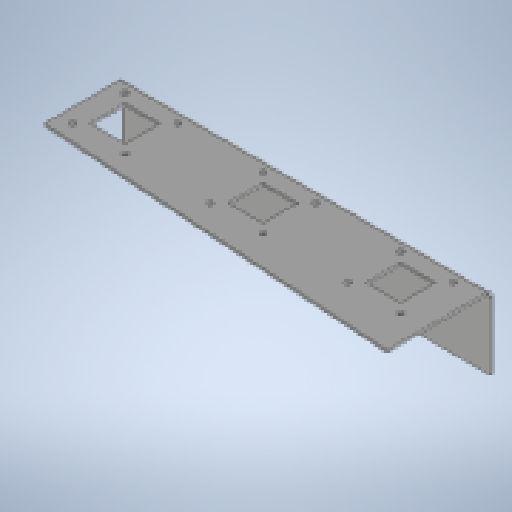
# Autodesk Inventor part: SLM 1422 BOTTOM FDS diameter way up
Saved by Autodesk Inventor 2026.2 (Build 302298000, 298)
## iProperties
Created: 2024-12-09
Part Number: SLM 1422 BOTTOM FDS diameter way up
Material: Stainless Steel
Document SubType Name: Sheet Metal
Designer: user
Mass: 793.765 g
Surface Area: 1023.32 cm^2
Volume: 99.2206 cm^3
Density: 8 g/cm^3
Flat Pattern Width: 15.2202 cm
Flat Pattern Length: 32 cm
Flat Pattern Area: 487.046 cm^2
Sheet Metal Rule: AISI304 2mm Die16
Sheet Metal Width: 152,202 mm
Sheet Metal Length: 320,000 mm
Sheet Metal Area: 48704,637 mm^2
Appearance: Default
Main_way_hight: 100,000 mm
Main_way_lenth: 410,000 mm
Small_ways_cross_H: 30,000 mm
Small_ways_cross_W: 30,000 mm
Author: user
Autodesk Inventor part; units mm, degrees
ref_plane "YZ Plane" through (0, 0, 0) normal (1, 0, 0) x (0, 1, 0)
ref_plane "XZ Plane" through (0, 0, 0) normal (0, 1, 0) x (-1, 0, 0)
ref_plane "XY Plane" through (0, 0, 0) normal (0, 0, 1) x (1, 0, 0)
sketch "Sketch1" plane through (0, 0, 0) normal (0, 0, 1) x (1, 0, 0)
  line L0 (0, 0) -> (-320, 0)
  line L1 (0, -92) -> (0, 0)
  line L2 (-320, 0) -> (-320, -70)
  line L3 (-320, -70) -> (0, -92)
  point P0 (0, -46)
  dimension "d32" = 92
  dimension "d60" = 70
  dimension "d61" = 320
  measures "d32" distance of L1.start L0.start
  measures "d60" distance of L0.end L2.end
  measures "d61" distance between parallel lines of L1 L2
extrude "Plate1" add sketch "Sketch1" along normal blind 2
sketch "Sketch8" plane through (0, 0, 2) normal (0, 0, 1) x (1, 0, 0)
  line L0 (-29.75, -50.25) -> (-60.25, -50.25)
  line L1 (-60.25, -50.25) -> (-60.25, -19.75)
  line L2 (-60.25, -19.75) -> (-29.75, -19.75)
  line L3 (-29.75, -19.75) -> (-29.75, -50.25)
  line L4 (-29.75, -50.25) -> (-60.25, -19.75) construction
  line L5 (-60.25, -50.25) -> (-29.75, -19.75) construction
  circle A0 centre (-22, -58) radius 2.5
  circle A1 centre (-68, -58) radius 2.5
  circle A2 centre (-68, -12) radius 2.5
  circle A3 centre (-22, -12) radius 2.5
  line L6 (0, 0) -> (0, -92) projected
  line L7 (-320, 0) -> (0, 0) projected
  line L8 (-60.25, -50.25) -> (-68, -58) construction
  line L9 (-68, -12) -> (-22, -12) construction
  line L10 (-22, -12) -> (-22, -58) construction
  line L11 (-22, -58) -> (-68, -58) construction
  line L12 (-68, -58) -> (-68, -12) construction
  point P0 (-45, -35)
  dimension "d51" = 30.5
  dimension "d52" = 30.5
  dimension "d53" = 5
  dimension "d72" = 45
  dimension "d78" = 46
  dimension "d79" = 12
  constraints: 22 end point, 4 centre point, 4 parallel, 4 point on line, 3 equal radius, 2 horizontal, 2 midpoint, 2 perpendicular
  measures "d51" distance of L0.start L0.end
  measures "d52" distance of L0.end L1.end
  measures "d53" diameter of A0
  measures "d72" distance from line of L6 point (-45, -35)
  measures "d78" distance of L8.end L9.start
  measures "d79" distance between parallel lines of L9 L7
extrude "Cut3" cut sketch "Sketch8" against normal blind 2
pattern_linear "Rectangular Pattern1" count 3 spacing 120 along (-1, 0, 0) of "Cut3"
sketch "Sketch9" plane through (0, -2, 2) normal (0, 1, 0) x (-1, 0, 0)
  line L0 (320, 0) -> (0, 0)
  line L1 (0, 0) -> (0, -64)
  line L2 (0, -64) -> (320, -64)
  line L3 (320, -64) -> (320, 0)
  constraints: 6 end point, 1 horizontal, 1 perpendicular, 1 vertical
edge flange "Flange3" height 64 angle 90 thickness 2 bend radius 2.75 thickness toward (0, 1, 0) relief round relief width 2 relief depth 1 edges at (-160, 0, 0) wall of the first edge with corners at (-320, -2, 2) (0, -2, 2) (0, -2, -62) (-320, -2, -62)
bend "Bend3"
corner "Corner3"
equation "\"d51\" = d52"
equation "\"d55\" = Thickness"
equation "\"d2\" = Thickness"
equation "\"d62\" = BendReliefWidth"
equation "\"d63\" = BendReliefDepth"
equation "\"d64\" = MinimumRemnant"
equation "\"d65\" = TransitionRadius"
equation "\"d66\" = MAIN_7_central_window_width + 2 * Thickness"
equation "\"d68\" = BendRadius"
equation "\"d69\" = CornerReliefSize"
equation "\"d70\" = GapSize"
equation "\"d71\" = JacobiRadiusSize"
equation "\"BendReliefWidth\" = Thickness"
equation "\"BendReliefDepth\" = 0.5 * Thickness"
equation "\"CornerReliefSize\" = 4 * Thickness"
equation "\"MinimumRemnant\" = 2 * Thickness"
equation "\"TransitionRadius\" = BendRadius"
equation "\"JacobiRadiusSize\" = BendRadius"
equation "\"GapSize\" = Thickness"
equation "\"Thickness\" = 2"
equation "\"MAIN_7_central_window_width\" = 60"
equation "\"BendRadius\" = 2.75"
body "Solid1"
